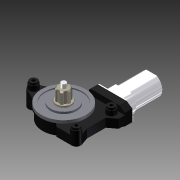
# Autodesk Inventor part: 262190-3030
Saved by Autodesk Inventor 2014 (Build 180170000, 170)
## iProperties
Category: Motors
Company: Autodesk, Inc.
Created: 2013-12-23
Part Number: 262190-3030
Document SubType Name: Modeling
Density: 2.17394 g/cm^3
Project: FIRST
Description: Motor - Denso Window Right
Vendor: Denso
Mass: 465 g
Surface Area: 382.475 cm^2
Volume: 213.897 cm^3
Material: Generic
Appearance: Glossy - Black
Title: Motor - Denso Window
Author: Autodesk, Inc.
Autodesk Inventor part; units mm, degrees
ref_plane "YZ Plane" through (0, 0, 0) normal (1, 0, 0) x (0, 1, 0)
sketch "Sketch1" plane through (0, 0, 0) normal (0, 0, 1) x (1, 0, 0)
  circle A0 centre (0, 0) radius 36
  circle A1 centre (0, 0) radius 30
  circle A2 centre (0, 0) radius 21
  circle A3 centre (0, 0) radius 12.9
  dimension "d0" = 72
  dimension "d3" = 60
  dimension "d4" = 42
  dimension "d5" = 25.8
  constraints: 4 centre point, 4 coincident
  measures "d0" diameter of A0
  measures "d3" diameter of A1
  measures "d4" diameter of A2
  measures "d5" diameter of A3
extrude "Extrusion1" add sketch "Sketch1" against normal blind 4.8 contours A0 | A1 | A2 | A3
extrude "Extrusion2" cut sketch "Sketch1" against normal blind 1.9 contours A1
extrude "Extrusion3" add sketch "Sketch1" along normal blind 1.2 contours A2
sketch "Sketch2" plane through (0, 0, 0) normal (0, 0, 1) x (1, 0, 0)
  circle A0 centre (0, 0) radius 12.9 projected
  circle A1 centre (0, 0) radius 11.9
  dimension "d10" = 23.8
  constraints: 1 centre point, 1 coincident
  measures "d10" diameter of A1
extrude "Extrusion4" add sketch "Sketch2" along normal blind 3 contours A1
sketch "Sketch3" plane through (0, 0, 3) normal (0, 0, 1) x (1, 0, 0)
  circle A0 centre (0, 0) radius 11.9 projected
  circle A1 centre (0, 0) radius 8.2
  dimension "d13" = 16.4
  constraints: 1 centre point, 1 coincident
  measures "d13" diameter of A1
extrude "Extrusion5" add sketch "Sketch3" along normal blind 18 contours A1
sketch "Sketch4" plane through (0, 0, 21) normal (0, 0, 1) x (1, 0, 0)
  circle A0 centre (0, 0) radius 8.2 projected
  circle A1 centre (0, 0) radius 4
  dimension "d16" = 8
  constraints: 1 centre point, 1 coincident
  measures "d16" diameter of A1
extrude "Extrusion6" add sketch "Sketch4" along normal blind 6.7 contours A1
sketch "Sketch5" plane through (0, 0, 21) normal (0, 0, 1) x (1, 0, 0)
  circle A0 centre (0, 0) radius 8.2 projected
  arc A1 (2, 9.7469) -> (-2, 9.7469) centre (0, 0) ccw
  line L0 (-2, 7.9524) -> (-2, 9.7469)
  line L1 (2, 7.9524) -> (2, 9.7469)
  dimension "d19" = 19.9
  dimension "d20" = 4
  constraints: 4 end point, 4 point on circle, 2 parallel, 1 centre point, 1 coincident, 1 vertical
  measures "d19" diameter of A1
  measures "d20" distance between parallel lines of L1 L0
extrude "Extrusion7" add sketch "Sketch5" against normal up to surface (18 mm away) contours A0 L0 A1 L1
chamfer "Chamfer1" distance 1.75 angle 45 1 edges at (0, 9.95, 21)
pattern_circular "Circular Pattern1" count 6 over 360 about axis through (0, 0, 3) along (0, 0, 1) of "Extrusion7", "Chamfer1"
sketch "Sketch6" plane through (0, 0, -4.8) normal (0, 0, -1) x (-1, 0, 0)
  circle A0 centre (0, 0) radius 36 projected
  circle A1 centre (0, 0) radius 34
  circle A2 centre (0, 48.7258) radius 7.1
  circle A3 centre (-28.38, -48.7258) radius 7.1
  circle A4 centre (28.38, -48.7258) radius 7.1
  line L0 (0, 48.7258) -> (-28.38, -48.7258) construction
  line L1 (-28.38, -48.7258) -> (28.38, -48.7258) construction
  line L2 (28.38, -48.7258) -> (0, 48.7258) construction
  line L3 (0, 48.7258) -> (0, -48.7258)
  circle A5 centre (0, 48.7258) radius 8.15
  line L4 (-18.5, 28.5263) -> (-7.3758, 52.1928)
  line L5 (18.5, 28.5263) -> (7.3758, 52.1928)
  line L6 (29.1893, -17.4351) -> (35.48, -23.7258)
  line L7 (35.48, -23.7258) -> (35.48, -48.7258)
  line L8 (13.5739, -51.0558) -> (26.0296, -55.4255)
  line L9 (13.5739, -51.0558) -> (-16.9261, -51.0558)
  line L10 (-16.9261, -51.0558) -> (-26, -63)
  line L11 (-26, -63) -> (-36, -63)
  line L12 (-36, -63) -> (-36, 0)
  line L13 (-36, 0) -> (-34, 0)
  dimension "d29" = 68
  dimension "d30" = 14.2
  dimension "d31" = 101.5
  dimension "d32" = 56.76
  dimension "d33" = 16.3
  dimension "d34" = 37
  dimension "d35" = 135
  dimension "d36" = 25
  dimension "d37" = 10
  dimension "d38" = 63
  dimension "d39" = 30.5
  dimension "d40" = 13.2
  dimension "d41" = 15
  constraints: 28 end point, 8 point on circle, 5 centre point, 4 tangent, 3 coincident, 3 perpendicular, 3 vertical, 2 equal radius, 2 midpoint, 2 vertical alignment, 1 equal length, 1 horizontal, 1 horizontal alignment, 1 parallel, 1 other
  measures "d29" diameter of A1
  measures "d30" diameter of A3
  measures "d31" distance of L0.start L0.end
  measures "d32" distance of L0.end L1.end
  measures "d33" diameter of A5
  measures "d34" distance of L5.start L4.start
  measures "d35" angle of L7 L6
  measures "d36" distance of L6.end L7.end
  measures "d37" distance of L10.end L11.end
  measures "d38" distance of L11.end L12.end
  measures "d39" distance of L8.start L9.end
  measures "d40" distance of L8.start L8.end
  measures "d41" distance of L9.end L10.end
extrude "Extrusion8" add sketch "Sketch6" along normal blind 18.6 contours A1 L3 | L3 A1
ref_plane "Work Plane1" through (0, 0, 6) normal (0, 0, 1) x (1, 0, 0)
extrude "Extrusion9" add sketch "Sketch6" along normal blind 17 contours L5 A1 L3 A0 | A0 L3 A5 L5 | L3 A1 L4 A0 | A0 L4 A5 L3 | A5 | A2
extrude "Extrusion10" add sketch "Sketch6" along normal blind 14 contours L6 L7 A4 L8 L9 L10 L11 L12 A0 | A0 L3 A1 L6 | A0 L13 A1 L3 | A4 | A3
sketch "Sketch7" plane through (0, 0, -23.4) normal (0, 0, -1) x (-1, 0, 0)
  circle A0 centre (0, 0) radius 34 projected
  circle A1 centre (0, 0) radius 9.75
  dimension "d49" = 19.5
  constraints: 1 centre point, 1 coincident
  measures "d49" diameter of A1
extrude "Extrusion11" [suppressed]
sketch "Sketch15" plane through (0, 0, 0) normal (1, 0, 0) x (0, 1, 0)
  line L0 (34, -23.4) -> (-34, -23.4) projected
  line L1 (-34, -23.4) -> (-9.8, -27.2)
  line L2 (-9.8, -27.2) -> (0, -27.2)
  line L3 (0, -23.4) -> (0, -27.2)
  point P0 (0, 0)
  dimension "d106" = 19.6
  dimension "d107" = 3.8
  constraints: 6 end point, 1 midpoint, 1 parallel, 1 perpendicular
  measures "d106" diameter of L1.end L3
  measures "d107" distance of L3.start L2.end
revolve "Revolution1" add sketch "Sketch15" angle 360 about axis through (0, 0, -23.4) along (0, 0, -1)
sketch "Sketch16" plane through (0, 0, -27.2) normal (0, 0, -1) x (-1, 0, 0)
  circle A0 centre (0, 0) radius 9.8 projected
  circle A1 centre (0, 0) radius 34 projected
  line L0 (0, 9.8) -> (0, 34)
  line L1 (-4.9, 8.487) -> (-17, 29.4449)
  arc A2 (0, 9.8) -> (-4.9, 8.487) centre (0, 0) ccw
  arc A3 (0, 34) -> (-17, 29.4449) centre (0, 0) ccw
  line L2 (0, 0) -> (-4.9, 8.487) construction
  line L3 (-15.6264, 29.0657) -> (-4.0084, 8.9427)
  line L4 (-1, 9.7488) -> (-1, 32.9848)
  arc A4 (-1, 32.9848) -> (-15.6264, 29.0657) centre (0, 0) ccw
  arc A5 (-1, 18.9737) -> (-8.6208, 16.9317) centre (0, 0) ccw
  arc A6 (-1, 20.9762) -> (-9.6221, 18.6659) centre (0, 0) ccw
  dimension "d109" = 30
  dimension "d110" = 1
  dimension "d111" = 19
  dimension "d112" = 2
  dimension "d113" = 1
  constraints: 18 point on circle, 10 end point, 5 centre point, 4 point on line, 2 coincident, 2 concentric, 1 collinear, 1 parallel, 1 vertical, 1 vertical alignment, 1 other
  measures "d109" angle of L1 L0
  measures "d110" distance between parallel lines of L0 L4
  measures "d111" radius of A5
  measures "d112" radial gap between concentric circles of A5 A6
  measures "d113" distance between parallel lines of L1 L3
extrude "Extrusion20" cut sketch "Sketch16" against normal blind 4.5 contours A0 L3 A5 L4 | A6 L3 A4 L4
pattern_circular "Circular Pattern2" count 12 over 360 about axis through (0, 0, -4.8) along (0, 0, -1) of "Extrusion20"
extrude "Extrusion12" add sketch "Sketch6" against normal up to surface (10.8 mm away) contours A4 | A2 | A3
sketch "Sketch10" plane through (0, 48.7258, 6) normal (0, 0, 1) x (1, 0, 0)
  circle A0 centre (0, 0) radius 7.1 projected
  circle A1 centre (0, 0) radius 5.95
  circle A2 centre (28.38, -97.4517) radius 7.1 projected
  circle A3 centre (-28.38, -97.4517) radius 7.1 projected
  circle A4 centre (28.38, -97.4517) radius 5.95
  circle A5 centre (-28.38, -97.4517) radius 5.95
  point P0 (0, -48.7258)
  dimension "d61" = 11.9
  constraints: 3 centre point, 3 coincident, 2 equal radius
  measures "d61" diameter of A1
extrude "Extrusion13" cut sketch "Sketch10" against normal blind 3
sketch "Sketch11" plane through (0, 48.7258, 6) normal (0, 0, 1) x (1, 0, 0)
  circle A0 centre (0, 0) radius 5.95 projected
  circle A1 centre (28.38, -97.4517) radius 5.95 projected
  circle A2 centre (-28.38, -97.4517) radius 5.95 projected
  point P0 (0, -48.7258)
hole "Hole2" at (0, 48.7258, 6) at (28.38, -48.7258, 6) at (-28.38, -48.7258, 6) direction (0, 0, -1) diameter 5 end through all
ref_plane "Work Plane4" through (0, 0, -30.2) normal (0, 0, 1) x (1, 0, 0)
sketch "Sketch14" plane through (0, 0, -21.8) normal (0, 0, -1) x (-1, 0, 0)
  circle A0 centre (0, 48.7258) radius 2.5 projected
  arc A1 (7.3758, 52.1928) -> (-7.3758, 52.1928) centre (0, 48.7258) ccw projected
  circle A2 centre (0, 48.7258) radius 8.15
  constraints: 1 centre point, 1 coincident, 1 concentric
extrude "Extrusion19" add sketch "Sketch14" along normal up to surface (8.4 mm away)
ref_plane "Work Plane2" through (0, -34, -4.8) normal (0, 1, 0) x (-1, 0, 0)
ref_plane "Work Plane3" through (0, 0, -11) normal (0, 0, 1) x (1, 0, 0)
sketch "Sketch12" plane through (36, -63, -4.8) normal (1, 0, 0) x (0, 0, -1)
  line L0 (-9.3, 58) -> (21.7, 58)
  line L1 (21.7, 58) -> (21.7, 0)
  line L2 (21.7, 0) -> (-9.3, 0)
  line L3 (-9.3, 0) -> (-9.3, 58)
  line L4 (0, 0) -> (14, 0) projected
  point P0 (-4.8, 63)
  point P1 (6.2, 29)
  point P2 (6.2, 0)
  point P3 (21.7, 29)
  dimension "d73" = 31
  constraints: 8 end point, 2 midpoint, 2 parallel, 1 collinear, 1 horizontal, 1 horizontal alignment, 1 perpendicular, 1 vertical alignment
  measures "d73" distance of L1.end L2.end
extrude "Extrusion14" add sketch "Sketch12" along normal blind 12
chamfer "Chamfer2" distance 6 distance2 9 1 edges at (42, -63, -26.5) measured on face at (44, -63, -8.9333)
chamfer "Chamfer3" distance 6 distance2 9 1 edges at (42, -63, 4.5) measured on face at (44, -63, -6.9333)
fillet "Fillet1" radius 3.75 2 edges at (42, -5, 4.5) (42, -5, -26.5)
sketch "Sketch13" plane through (48, -63, -4.8) normal (1, 0, 0) x (0, 0, -1)
  line L0 (21.7, 58) -> (21.7, 0) projected
  line L1 (-9.3, 0) -> (-9.3, 58) projected
  line L2 (21.7, 0) -> (-9.3, 0) projected
  arc A0 (-9.1, 16.1972) -> (21.5, 16.1972) centre (6.2, 29) ccw
  arc A1 (21.5, 41.8028) -> (-9.1, 41.8028) centre (6.2, 29) ccw
  arc A2 (-9.1, 11.8941) -> (5.1507, 6.074) centre (6.2, 29) ccw
  line L3 (21.7, 9) -> (15.7, 0) projected
  line L4 (-3.3, 0) -> (-9.3, 9) projected
  line L5 (21.7, 9) -> (15.7, 0)
  line L6 (9.2, 0) -> (5.1507, 6.074)
  arc A3 (-5.55, 58) -> (-9.3, 54.25) centre (-5.55, 54.25) ccw projected
  arc A4 (21.7, 54.25) -> (17.95, 58) centre (17.95, 54.25) ccw projected
  arc A5 (-9.1, 20.6088) -> (21.5, 20.6088) centre (6.2, 29) ccw
  arc A6 (21.5, 37.3912) -> (-9.1, 37.3912) centre (6.2, 29) ccw
  circle A7 centre (6.2, 29) radius 5
  line L7 (-5.55, 57.8) -> (17.95, 57.8)
  line L8 (21.5, 54.25) -> (21.5, 8.7)
  line L9 (-9.1, 11.8941) -> (-9.1, 54.25)
  arc A8 (-5.55, 57.8) -> (-9.1, 54.25) centre (-5.55, 54.25) ccw
  arc A9 (21.5, 54.25) -> (17.95, 57.8) centre (17.95, 54.25) ccw
  line L10 (15.8333, 0.2) -> (9.0667, 0.2)
  point P0 (-4.8, 63)
  point P1 (6.2, 0)
  point P2 (21.7, 29)
  point P3 (-9.3, 16.44)
  point P4 (21.7, 16.44)
  point P5 (21.7, 41.56)
  point P6 (-9.3, 37.0158)
  point P7 (-9.3, 20.9842)
  point P8 (21.7, 20.9842)
  point P9 (21.7, 37.0158)
  dimension "d84" = 6.5
  dimension "d86" = 19.95
  dimension "d89" = 17.45
  dimension "d90" = 3
  dimension "d91" = 10
  dimension "d100" = 0.2
  dimension "d101" = 3.55
  constraints: 15 point on line, 14 point on circle, 12 end point, 8 centre point, 4 tangent, 3 equal radius, 2 coincident, 1 collinear, 1 horizontal alignment, 1 midpoint, 1 parallel, 1 vertical alignment, 6 other
  measures "d84" distance of L6.start L3.end
  measures "d86" radius of A1
  measures "d89" radius of A6
  measures "d90" radial gap between concentric circles of A2 A0
  measures "d91" diameter of A7
  measures "d100" distance between parallel lines of L9 L1
  measures "d101" radius of A8
extrude "Extrusion15" add sketch "Sketch13" along normal blind 2 contours L3 L10 L6 A2 L9 A0 L8 | A0 L9 A5 L8 | A5 L9 A6 L8 | A6 L9 A1 L8 | A1 L9 A8 L7 A9 L8 | A7
extrude "Extrusion16" add sketch "Sketch13" along normal blind 15 contours A0 L9 A5 L8 | A5 L9 A6 L8 | A6 L9 A1 L8 | A7
extrude "Extrusion17" add sketch "Sketch13" along normal blind 60 contours A5 L9 A6 L8 | A7
extrude "Extrusion18" add sketch "Sketch13" along normal blind 67 contours A7
body "Solid1"
